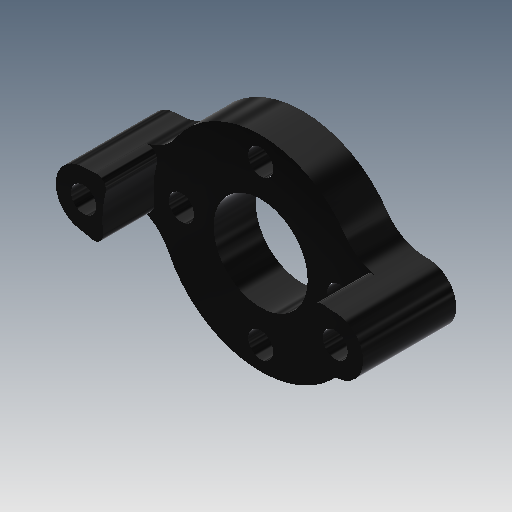
# Autodesk Inventor part: ジグ_1_1
Saved by Autodesk Inventor 2017.3 (Build 213256000, 256)
## iProperties
Created: 2016-05-31
Part Number: ジグ_1_1
Material: アセタール樹脂、黒
Document SubType Name: Modeling
Designer: hiroaki
Density: 1.425 g/cm^3
Appearance: 滑らか - 黒
Mass: 2.46976 g
Surface Area: 17.256 cm^2
Volume: 1.73317 cm^3
Author: hiroaki
Autodesk Inventor part; units mm, degrees
ref_plane "YZ Plane" through (0, 0, 0) normal (1, 0, 0) x (0, 1, 0)
ref_plane "XZ Plane" through (0, 0, 0) normal (0, 1, 0) x (-1, 0, 0)
ref_plane "XY Plane" through (0, 0, 0) normal (0, 0, 1) x (1, 0, 0)
sketch "スケッチ1" plane through (0, 0, 0) normal (0, 0, 1) x (1, 0, 0)
  circle A0 centre (0, 0) radius 11 construction
  circle A1 centre (0, 8.5) radius 1.35
  circle A2 centre (-8.5, 0) radius 1.35
  circle A3 centre (0, -8.5) radius 1.35
  circle A4 centre (8.5, 0) radius 1.35
  circle A5 centre (0, 0) radius 5.05
  circle A6 centre (-13.5, 1) radius 1.35
  circle A7 centre (13.5, 1) radius 1.35
  line L0 (-13.5, 15.0392) -> (13.5, 15.0392) construction
  line L1 (13.5, 15.0392) -> (13.5, 1) construction
  line L2 (13.5, 1) -> (-13.5, 1) construction
  line L3 (-13.5, 1) -> (-13.5, 15.0392) construction
  line L4 (-13.5, 4) -> (-10.247, 4)
  arc A8 (-13.5, 4) -> (-13.5, -2) centre (-13.5, 1) ccw
  line L5 (-13.5, -2) -> (-10.8167, -2)
  arc A9 (10.247, 4) -> (-10.247, 4) centre (0, 0) ccw
  arc A10 (-10.8167, -2) -> (10.8167, -2) centre (0, 0) ccw
  line L6 (10.247, 4) -> (13.5, 4)
  line L7 (10.8167, -2) -> (13.5, -2)
  arc A11 (13.5, -2) -> (13.5, 4) centre (13.5, 1) ccw
  point P0 (0, 15.0392)
  dimension "d0" = 22
  dimension "d1" = 2.7
  dimension "d2" = 8.5
  dimension "d5" = 360
  dimension "d7" = 10.1
  dimension "d8" = 2.7
  dimension "d9" = 27
  dimension "d10" = 1
  dimension "d11" = 3
  constraints: 16 end point, 12 centre point, 12 point on circle, 5 coincident, 5 tangent, 4 equal radius, 4 horizontal, 2 parallel, 2 perpendicular, 2 vertical alignment, 1 midpoint, 9 other
  measures "d0" diameter of A0
  measures "d1" diameter of A1
  measures "d2" distance of point (0, 0) A1.centre
  measures "d7" diameter of A5
  measures "d8" diameter of A7
  measures "d9" distance of L1.end L2.end
  measures "d10" distance from line of point (0, 0) L2
  measures "d11" radius of A8
extrude "押し出し1" add sketch "スケッチ1" along normal blind 10
sketch "スケッチ2" plane through (0, 0, 10) normal (0, 0, 1) x (1, 0, 0)
  circle A0 centre (0, 0) radius 5.05 projected
  circle A1 centre (8.5, 0) radius 1.35 projected
  circle A2 centre (0, -8.5) radius 1.35 projected
  circle A3 centre (-8.5, 0) radius 1.35 projected
  circle A4 centre (0, 8.5) radius 1.35 projected
  arc A5 (10.247, 4) -> (-10.247, 4) centre (0, 0) ccw projected
  circle A6 centre (0, 0) radius 11.5
  dimension "d14" = 0.5
  constraints: 1 centre point, 1 coincident
  measures "d14" radial gap between concentric circles of A6 A5
extrude "押し出し2" cut sketch "スケッチ2" against normal blind 5.5
fillet "フィレット1" radius 5 4 edges at (10.8167, -2, 2.25) (-10.8167, -2, 2.25) (-10.247, 4, 2.25) (10.247, 4, 2.25)
fillet "フィレット2" radius 1 5 edges at (-10.4214, 4.8625, 7.25) (-11.0252, -3.2702, 7.25) (10.4214, 4.8625, 7.25) (11.4684, 0.8515, 4.5) (11.0252, -3.2702, 7.25)
